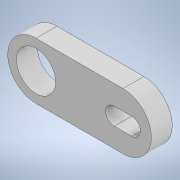
# Autodesk Inventor part: ChainLinkEnd
Saved by Autodesk Inventor 2020 (Build 240168000, 168)
## iProperties
Created: 2020-01-19
Part Number: ChainLinkEnd
Material: Generic
Document SubType Name: Modeling
Designer: srini
Density: 1 g/cm^3
Appearance: Default
Author: srini
Autodesk Inventor part; units mm, degrees
ref_plane "YZ Plane" through (0, 0, 0) normal (1, 0, 0) x (0, 1, 0)
ref_plane "XZ Plane" through (0, 0, 0) normal (0, 1, 0) x (-1, 0, 0)
ref_plane "XY Plane" through (0, 0, 0) normal (0, 0, 1) x (1, 0, 0)
sketch "Sketch1" plane through (0, 0, 0) normal (0, 0, 1) x (1, 0, 0)
  line L0 (31.75, 0) -> (-31.75, 0) construction
  line L1 (31.75, 20.6502) -> (-31.75, 20.6502)
  line L2 (-31.75, -20.6502) -> (31.75, -20.6502)
  arc A0 (31.75, -20.6502) -> (31.75, 20.6502) centre (31.75, 0) ccw
  arc A1 (-31.75, 20.6502) -> (-31.75, -20.6502) centre (-31.75, 0) ccw
  point P0 (0, 0)
  dimension "d0" = 20.6502
  dimension "d1" = 63.5
  constraints: 8 end point, 4 point on circle, 4 tangent, 2 centre point, 1 horizontal, 1 midpoint, 1 parallel
  measures "d0" radius of A1
  measures "d1" distance of L0.start L0.end
extrude "Extrusion1" add sketch "Sketch1" along normal blind 15.24
sketch "Sketch2" plane through (0, 0, 15.24) normal (0, 0, 1) x (1, 0, 0)
  arc A0 (-31.75, 20.6502) -> (-31.75, -20.6502) centre (-31.75, 0) ccw projected
  circle A1 centre (-31.75, 0) radius 14.3002
  line L0 (38.1, 0) -> (25.4, 0) construction
  line L1 (38.1, 6.35) -> (25.4, 6.35)
  line L2 (25.4, -6.35) -> (38.1, -6.35)
  arc A2 (38.1, -6.35) -> (38.1, 6.35) centre (38.1, 0) ccw
  arc A3 (25.4, 6.35) -> (25.4, -6.35) centre (25.4, 0) ccw
  point P0 (0, 0)
  point P1 (31.75, 0)
  dimension "d4" = 28.6004
  dimension "d5" = 12.7
  dimension "d6" = 6.35
  dimension "d7" = 25.4
  constraints: 8 end point, 4 point on circle, 4 tangent, 3 centre point, 1 coincident, 1 horizontal, 1 midpoint, 1 parallel, 1 point on line
  measures "d4" diameter of A1
  measures "d5" distance of L0.start L0.end
  measures "d6" radius of A3
  measures "d7" distance of L0.end point (0, 0)
extrude "Extrusion2" cut sketch "Sketch2" against normal through all
body "Solid1"
